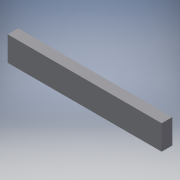
# Autodesk Inventor part: Tun-Brace
Saved by Autodesk Inventor 2017 (Build 210142000, 142)
## iProperties
Created: 2017-08-30
Part Number: Tun-Brace
Material: Generic
Document SubType Name: Modeling
Designer: Trent
Density: 1 g/cm^3
Appearance: Yellow Pine - Solid Stained Light Low Gloss
Author: Trent
Autodesk Inventor part; units mm, degrees
ref_plane "YZ Plane" through (0, 0, 0) normal (1, 0, 0) x (0, 1, 0)
ref_plane "XZ Plane" through (0, 0, 0) normal (0, 1, 0) x (-1, 0, 0)
ref_plane "XY Plane" through (0, 0, 0) normal (0, 0, 1) x (1, 0, 0)
sketch "Sketch1" plane through (0, 0, 0) normal (0, 0, 1) x (1, 0, 0)
  line L0 (-269.875, -44.45) -> (269.875, -44.45)
  line L1 (269.875, -44.45) -> (269.875, 44.45)
  line L2 (269.875, 44.45) -> (-269.875, 44.45)
  line L3 (-269.875, 44.45) -> (-269.875, -44.45)
  line L4 (-269.875, -44.45) -> (269.875, 44.45) construction
  line L5 (269.875, -44.45) -> (-269.875, 44.45) construction
  point P0 (0, 0)
  dimension "d0" = 539.75
  dimension "d1" = 88.9
  constraints: 12 end point, 2 midpoint, 2 parallel, 1 horizontal, 1 perpendicular
  measures "d0" distance of L2.end L1.end
  measures "d1" distance of L1.end L0.end
extrude "Extrusion1" add sketch "Sketch1" along normal blind 19.05
body "Solid1"
